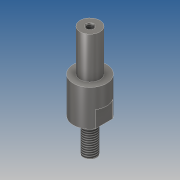
# Autodesk Inventor part: 200-60-DIFFERENTIAL-CONNECTOR-02
Saved by Autodesk Inventor 2018.2 (Build 222227000, 227)
## iProperties
Manager: feesmrt
Company: FRANC0R
Created: 2017-12-05
Part Number: 200-60-DIFFERENTIAL-CONNECTOR-02
Material: Edelstahl
Document SubType Name: Modeling
Designer: feesmrt
Density: 8 g/cm^3
Appearance: Halbpoliert
Project: Rescue Robot
Cost Center: -
Engineer: feesmrt
Authority: feesmrt
Description: Differential Connector
Stock Number: 200-60-DIFFERENTIAL-CONNECTOR-02
Author: feesmrt
Subject: Rescue Robot
Title: Differential Connector
Revision Number: 1
Autodesk Inventor part; units mm, degrees
ref_plane "YZ Plane" through (0, 0, 0) normal (1, 0, 0) x (0, 1, 0)
ref_plane "XZ Plane" through (0, 0, 0) normal (0, 1, 0) x (-1, 0, 0)
ref_plane "XY Plane" through (0, 0, 0) normal (0, 0, 1) x (1, 0, 0)
sketch "Skizze1" plane through (0, 0, 0) normal (1, 0, 0) x (0, 1, 0)
  line L0 (0, 38.36) -> (0, -55.16) projected
  line L1 (-2, 0) -> (12, 0) construction
  line L2 (6, 0) -> (6, 25)
  line L3 (6, 25) -> (0, 25)
  line L4 (6, 0) -> (10, 0)
  line L5 (10, 0) -> (10, -21.8)
  line L6 (10, -21.8) -> (4, -21.8)
  line L7 (4, -21.8) -> (4, -41.8)
  line L8 (4, -41.8) -> (0, -41.8)
  line L9 (0, -41.8) -> (0, 25)
  point P0 (0, 0)
  dimension "d0" = 12
  dimension "d1" = 25
  dimension "d3" = 8
  dimension "d4" = 21.8
  dimension "d6" = 20
  dimension "d23" = 20
  constraints: 16 end point, 5 perpendicular, 4 point on line, 2 vertical
  measures "d0" diameter of L2 L0
  measures "d1" distance between parallel lines of L1 L3
  measures "d3" diameter of L7 L0
  measures "d4" distance of L4.end L5.end
  measures "d6" diameter of L5 L0
  measures "d23" distance between parallel lines of L6 L8
revolve "Grundkörper" add sketch "Skizze1" angle 360 about axis through (0, 0, 0) along (0, 0, -1)
thread "M8" size "M8x1.25" class "6g" standard "ANSI Metric M Profile" full length
sketch "Skizze2" plane through (0, 0, 25) normal (0, 0, 1) x (1, 0, 0)
  circle A0 centre (0, 0) radius 6 projected
hole "M5x10" at (0, 0, 25) direction (0, 0, -1) diameter 4.134 depth 14.2 tip angle 118 countersink diameter 5 countersink angle 90 thread size "M5x0.8" class "6H" standard "ISO Metric profile"
sketch "Skizze3" plane through (0, 0, 0) normal (0, 1, 0) x (-1, 0, 0)
  line L0 (0, -24.96) -> (0, 4.16) construction
  line L1 (-10, -21.8) -> (10, -21.8) construction
  line L2 (10, 0) -> (10, -21.8) construction
  line L3 (-10, 0) -> (-10, -21.8) construction
  line L4 (8.5, -21.8) -> (8.5, -11.8)
  line L5 (8.5, -11.8) -> (10, -11.8)
  line L6 (10, -11.8) -> (10, -21.8)
  line L7 (10, -21.8) -> (8.5, -21.8)
  line L8 (-10, -11.8) -> (-8.5, -11.8)
  line L9 (-8.5, -11.8) -> (-8.5, -21.8)
  line L10 (-8.5, -21.8) -> (-10, -21.8)
  line L11 (-10, -21.8) -> (-10, -11.8)
  point P0 (0, 0)
  dimension "d24" = 10
  dimension "d25" = 17
  constraints: 16 end point, 6 point on line, 4 collinear, 3 perpendicular, 1 vertical
  measures "d24" distance of L4.start L4.end
  measures "d25" distance between parallel lines of L9 L4
extrude "Extrusion1" cut sketch "Skizze3" along normal through all both and the other way through all
